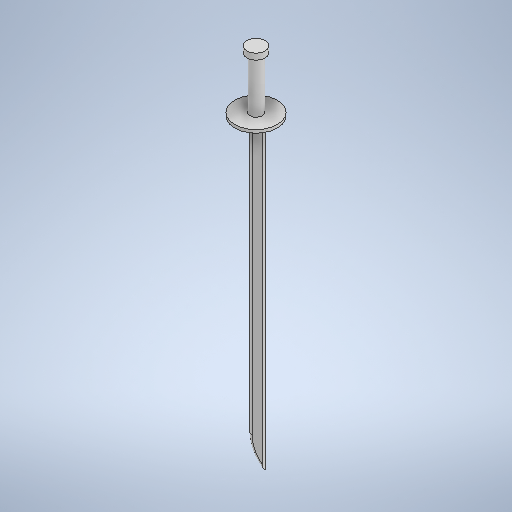
# Autodesk Inventor part: katana
Saved by Autodesk Inventor 2025.2 (Build 292293000, 293)
## iProperties
Created: 2025-03-25
Part Number: katana
Material: Genérico
Document SubType Name: Modeling
Designer: Carlos Dias
Density: 1 g/cm^3
Appearance: Padrão
Author: Carlos Dias
Autodesk Inventor part; units mm, degrees
ref_plane "YZ Plane" through (0, 0, 0) normal (1, 0, 0) x (0, 1, 0)
ref_plane "XZ Plane" through (0, 0, 0) normal (0, 1, 0) x (-1, 0, 0)
ref_plane "XY Plane" through (0, 0, 0) normal (0, 0, 1) x (1, 0, 0)
sketch "Esboço1" plane through (0, 0, 0) normal (0, 0, 1) x (1, 0, 0)
  line L0 (-3, 20) -> (0, 20)
  line L1 (-3, 20) -> (-3, 18)
  line L2 (-3, 18) -> (-2, 18)
  line L3 (-2, 18) -> (-2, 1)
  line L4 (-2, 1) -> (-7, 1)
  line L5 (-7, 1) -> (-7, 0)
  line L6 (-7, 0) -> (0, 0)
  line L7 (0, 20) -> (0, 0)
  line L8 (-8.4, 0) -> (1.4, 0) projected
  line L9 (0, -4) -> (0, 24) projected
  dimension "d0" = 20
  dimension "d1" = 3
  dimension "d2" = 2
  dimension "d3" = 1
  dimension "d4" = 5
  dimension "d5" = 1
  constraints: 16 end point, 3 horizontal, 3 vertical, 2 perpendicular, 1 vertical alignment
  measures "d0" distance from line of L6.end L0
  measures "d1" distance of L0.start L0.end
  measures "d2" distance of L0.start L1.end
  measures "d3" distance of L1.end L2.end
  measures "d4" distance of L3.end L4.end
  measures "d5" distance between parallel lines of L6 L4
revolve "Revolução1" add sketch "Esboço1" angle 360 about axis through (0, -10, 0) along (0, 1, 0)
sketch "Esboço2" plane through (0, 0, 0) normal (0, 0, 1) x (1, 0, 0)
  line L0 (-2.5, 0) -> (2.5, 0)
  line L1 (2.5, 0) -> (2.5, -100)
  line L2 (2.5, -100) -> (2.5, -64.1353)
  arc A0 (-2.5, -91.3397) -> (2.5, -100) centre (7.5, -91.3397) ccw
  line L3 (-2.5, 0) -> (-2.5, -91.3397)
  line L4 (7, 0) -> (-7, 0) projected
  point P0 (0, 0)
  point P1 (0, 0)
  dimension "d7" = 100
  dimension "d8" = 5
  dimension "d10" = 10
  constraints: 8 end point, 2 midpoint, 2 point on circle, 2 vertical, 1 centre point, 1 coincident, 1 horizontal, 1 point on line, 1 tangent
  measures "d7" distance of L0.end L1.end
  measures "d8" distance of L0.start L0.end
  measures "d10" radius of A0
extrude "Extrusão1" add sketch "Esboço2" along normal mid plane 1
fillet "Arredondamento1" radius 2 2 edges at (-1.1603, -96.3397, 0.5) (-2.5, -45.6699, 0.5)
